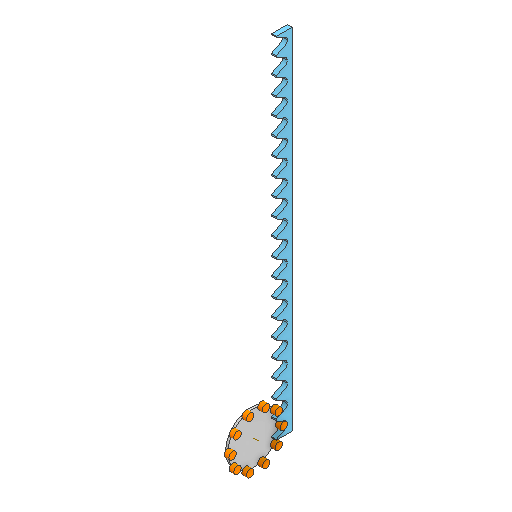
# Autodesk Inventor part: Trochoidal Rack
Saved by Autodesk Inventor 2025.3 (Build 293356000, 356)
## iProperties
Created: 2026-06-12
Part Number: Trochoidal Rack
Material: Generic
Document SubType Name: Modeling
Designer: PC
Density: 1 g/cm^3
Appearance: Default
Author: PC
Autodesk Inventor part; units mm, degrees
ref_plane "YZ Plane" through (0, 0, 0) normal (1, 0, 0) x (0, 1, 0)
ref_plane "XZ Plane" through (0, 0, 0) normal (0, 1, 0) x (-1, 0, 0)
ref_plane "XY Plane" through (0, 0, 0) normal (0, 0, 1) x (1, 0, 0)
sketch "Sketch1" plane through (0, 0, 0) normal (1, 0, 0) x (0, 1, 0)
  spline S0 degree 4 poles (0, -3) (2.996, -3.0108) (6.2199, -1.4987) (8.6151, 2.966) (10.4612, 7.4343) (12.4058, 11.8024) (14.5191, 16.0073) (15.9132, 18.5396) (17.3635, 21) knots 0 0 0 0 0 0.389779 0.389779 0.631316 0.631316 1 1 1 1 1
  circle A0 centre (0, 60) radius 55 construction
  circle A1 centre (0, 60) radius 60 construction
  line L0 (0, 60) -> (0, 5) construction
  line L1 (0, 5) -> (0, 0) construction
  circle A2 centre (0, 5) radius 8 construction
  line L2 (0, -13) -> (0, -3)
  line L3 (0, 60) -> (60, 60) construction
  line L4 (0, -3) -> (37.6991, -3) construction
  line L5 (17.3635, 21) -> (18.8496, 21)
  line L6 (18.8496, 21) -> (18.8496, -13)
  line L7 (18.8496, -13) -> (0, -13)
  point P0 (18.8496, -3)
  dimension "d4" = 110
  dimension "d5" = 120
  dimension "d6" = 16
  dimension "d20" = 10
  dimension "d70" = 37.6991
  constraints: 16 end point, 4 vertical, 3 coincident, 2 centre point, 2 horizontal, 2 point on circle, 2 vertical alignment, 1 midpoint, 1 perpendicular, 1 tangent, 5 other
  measures "d5" diameter of A1
  measures "d6" diameter of A2
  measures "d20" distance of L2.start L2.end
  measures "d70" distance of L2.end L4.end
extrude "Extrusion2" add sketch "Sketch1" along normal blind 10
mirror "Mirror1" about plane through (0, 0, 0) normal (0, 1, 0)
pattern_linear "Rectangular Pattern4" count 20 spacing 37.6991 along (0, 1, 0)
sketch "Sketch3" plane through (0, 0, 0) normal (-1, 0, 0) x (0, 0, 1)
  circle A0 centre (60, 0) radius 55 projected
  point P0 (0, 0)
extrude "Extrusion3" add sketch "Sketch3" along normal blind 5 separate body
sketch "Sketch4" plane through (0, 0, 0) normal (-1, 0, 0) x (0, 0, 1)
  circle A0 centre (5, 0) radius 8 projected
  point P0 (0, 0)
extrude "Extrusion4" add sketch "Sketch4" against normal blind 10 bodies 2
pattern_circular "Circular Pattern1" count 10 over 360 about axis through (0, 0, 60) along (-1, 0, 0) of "Extrusion4" bodies 2
equation "\"module\" = 11"
equation "\"d24\" = 55"
equation "\"d25\" = 1.454545"
equation "\"d26\" = 11"
equation "\"d27\" = 0.454545"
equation "\"d32\" = 55"
equation "\"d33\" = 1.454545"
equation "\"d34\" = 11"
equation "\"d35\" = 0.454545"
equation "\"d40\" = 55"
equation "\"d41\" = 1.454545"
equation "\"d42\" = 11"
equation "\"d43\" = 0.454545"
equation "\"d48\" = 55"
equation "\"d49\" = 1.454545"
equation "\"d50\" = 11"
equation "\"d51\" = 0.454545"
equation "\"d56\" = 55"
equation "\"d57\" = 1.454545"
equation "\"d58\" = 11"
equation "\"d59\" = 0.454545"
equation "curve S0 of \"Sketch1\": x = R*t-r*sin(t*180/PI)+r*sin(t*180/PI)*module*c_f/(2*sqrt((r*sin(t*180/PI))^2+(r*cos(t*180/PI)-R)^2)); y = R-r*cos(t*180/PI)+(r*cos(t*180/PI)-R)*module*c_f/(2*sqrt((r*sin(t*180"
body "Solid2"
body "Solid3"
